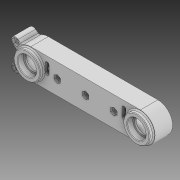
# Autodesk Inventor part: Scara1
Saved by Autodesk Inventor 2020 (Build 240168000, 168)
## iProperties
Created: 2020-07-24
Part Number: Scara1
Material: Generic
Document SubType Name: Modeling
Designer: DDeGo
Density: 1 g/cm^3
Appearance: Default
Author: DDeGo
Autodesk Inventor part; units mm, degrees
ref_plane "YZ Plane" through (0, 0, 0) normal (1, 0, 0) x (0, 1, 0)
ref_plane "XZ Plane" through (0, 0, 0) normal (0, 1, 0) x (-1, 0, 0)
ref_plane "XY Plane" through (0, 0, 0) normal (0, 0, 1) x (1, 0, 0)
sketch "Sketch1" plane through (0, 0, 0) normal (0, 0, 1) x (1, 0, 0)
  line L0 (0, 0) -> (97, 0) construction
  line L1 (0, -13) -> (97, -13)
  line L2 (97, 13) -> (0, 13)
  arc A0 (0, 13) -> (0, -13) centre (0, 0) ccw
  arc A1 (97, -13) -> (97, 13) centre (97, 0) ccw
  point P0 (48.5, 0)
  dimension "d0" = 97
  dimension "d1" = 13
  constraints: 8 end point, 4 point on circle, 4 tangent, 2 centre point, 1 horizontal, 1 midpoint, 1 parallel
  measures "d0" distance of L0.start L0.end
  measures "d1" radius of A0
extrude "Extrusion1" add sketch "Sketch1" along normal blind 3
sketch "Sketch2" plane through (0, 0, 0) normal (0, 0, -1) x (-1, 0, 0)
  line L0 (-97, 13) -> (0, 13) projected
  arc A0 (-97, 13) -> (-97, -13) centre (-97, 0) ccw projected
  line L1 (0, -13) -> (-97, -13) projected
  arc A1 (0, -13) -> (0, 13) centre (0, 0) ccw projected
  line L2 (0, 10) -> (-97, 10)
  arc A2 (-97, 10) -> (-97, -10) centre (-97, 0) ccw
  line L3 (-97, -10) -> (0, -10)
  arc A3 (0, -10) -> (0, 10) centre (0, 0) ccw
  point P0 (-94.4322, -13)
  dimension "d17" = 3
  constraints: 4 end point, 4 point on circle, 2 centre point, 1 point on line, 3 other
  measures "d17" distance between parallel lines of L2 L0
extrude "Extrusion2" add sketch "Sketch2" along normal blind 12.5
sketch "Sketch5" plane through (0, 0, 0) normal (0, 0, -1) x (-1, 0, 0)
  circle A0 centre (0, 0) radius 3
  arc A1 (-97, 13) -> (-97, -13) centre (-97, 0) ccw projected
  circle A2 centre (-97, 0) radius 3
  dimension "d14" = 6
  constraints: 2 centre point, 2 coincident, 1 equal radius
  measures "d14" diameter of A2
extrude "Extrusion5" cut sketch "Sketch5" against normal through all
sketch "Sketch6" plane through (0, 0, 3) normal (0, 0, 1) x (1, 0, 0)
  circle A0 centre (0, 0) radius 8.15
  circle A1 centre (0, 0) radius 11.65
  dimension "d18" = 16.3
  dimension "d19" = 3.5
  constraints: 2 centre point, 2 coincident
  measures "d18" diameter of A0
  measures "d19" radial gap between concentric circles of A1 A0
extrude "Extrusion6" add sketch "Sketch6" along normal blind 3.5
sketch "Sketch7" plane through (0, 0, 6.5) normal (0, 0, 1) x (1, 0, 0)
  circle A0 centre (0, 0) radius 8.15 projected
extrude "Extrusion7" cut sketch "Sketch7" against normal blind 5
chamfer "Chamfer1" distance 1 angle 45 1 edges at (-11.65, 0, 3)
sketch "Sketch8" plane through (0, 0, 1.5) normal (0, 0, 1) x (1, 0, 0)
  circle A0 centre (0, 0) radius 8.15 projected
  circle A1 centre (0, 0) radius 6.65
  dimension "d27" = 1.5
  constraints: 1 centre point
  measures "d27" radial gap between concentric circles of A0 A1
extrude "Extrusion8" cut sketch "Sketch8" against normal through all contours A1
sketch "Sketch9" plane through (0, 0, 0) normal (0, 0, -1) x (-1, 0, 0)
  circle A0 centre (-97, 0) radius 3 projected
  circle A1 centre (0, 0) radius 3 projected
  line L0 (-97, 0) -> (0, 0) construction
  circle A2 centre (-73.5, 0) radius 4
  circle A3 centre (-73.5, 0) radius 1.75
  circle A4 centre (-48.5, 0) radius 4
  circle A5 centre (-48.5, 0) radius 1.75
  circle A6 centre (-23.5, 0) radius 4
  circle A7 centre (-23.5, 0) radius 1.75
  dimension "d30" = 3.5
  dimension "d31" = 8
  dimension "d42" = 25
  dimension "d67" = 25
  constraints: 6 centre point, 4 equal radius, 3 coincident, 2 end point, 2 point on line, 1 horizontal, 1 midpoint
  measures "d30" diameter of A3
  measures "d31" diameter of A2
  measures "d42" distance of A4.centre A2.centre
  measures "d67" distance of A6.centre A4.centre
extrude "Extrusion9" add sketch "Sketch9" along normal up to surface (12.5 mm away) contours A2 | A4 | A6
sketch "Sketch10" plane through (0, 0, 0) normal (0, 1, 0) x (-1, 0, 0)
  line L0 (-69.5, 0) -> (-69.5, -12.5) projected
  line L1 (-52.5, 0) -> (-52.5, -12.5) projected
  line L2 (-44.5, 0) -> (-44.5, -12.5) projected
  line L3 (-27.5, 0) -> (-27.5, -12.5) projected
  line L4 (-69.5, -12.5) -> (-77.5, -12.5) projected
  line L5 (-69.5, -12.5) -> (-52.5, -12.5)
  line L6 (-44.5, -12.5) -> (-27.5, -12.5)
  line L7 (-44.5, 0) -> (-52.5, 0) projected
  line L8 (-27.5, 0) -> (-44.5, 0)
  line L9 (-69.5, 0) -> (-77.5, 0) projected
  line L10 (-52.5, 0) -> (-69.5, 0)
  line L11 (-69.5, -12.5) -> (-70.5, -12.5)
  line L12 (-70.5, -12.5) -> (-70.5, 0)
  line L13 (-69.5, 0) -> (-70.5, 0)
  line L14 (-44.5, -12.5) -> (-52.5, -12.5) projected
  line L15 (-52.5, -12.5) -> (-51.5, -12.5)
  line L16 (-51.5, -12.5) -> (-51.5, 0.1572)
  line L17 (-51.5, 0.1572) -> (-52.5, 0)
  line L18 (-44.5, 0) -> (-45.5, 0)
  line L19 (-44.5, -12.5) -> (-45.5, -12.5)
  line L20 (-45.5, -12.5) -> (-45.5, 0)
  line L21 (-27.5, -12.5) -> (-26.5, -12.5)
  line L22 (-26.5, -12.5) -> (-26.5, 0)
  line L23 (-19.5, 0) -> (-27.5, 0) projected
  line L24 (-26.5, 0) -> (-27.5, 0)
  line L25 (-27.5, 0) -> (-26.5, 0)
  circle A0 centre (-73.4335, -3.2498) radius 2
  circle A1 centre (-56.5768, -5.2498) radius 2
  circle A2 centre (-26.4602, -5.2498) radius 2
  circle A3 centre (-43.2818, -5.75) radius 2
  point P0 (0, 0)
  point P1 (-51.5, 0)
  dimension "d38" = 1
  dimension "d39" = 1
  dimension "d40" = 1
  dimension "d41" = 1
  dimension "d50" = 4
  dimension "d51" = 4
  dimension "d52" = 4
  dimension "d53" = 4
  constraints: 34 end point, 6 point on line, 5 perpendicular, 4 centre point, 4 collinear, 2 horizontal, 1 parallel
  measures "d38" distance between parallel lines of L3 L22
  measures "d39" distance between parallel lines of L2 L20
  measures "d40" distance between parallel lines of L1 L16
  measures "d41" distance between parallel lines of L0 L12
  measures "d50" diameter of A2
  measures "d51" diameter of A1
  measures "d52" diameter of A0
  measures "d53" diameter of A3
extrude "Extrusion10" add sketch "Sketch10" along normal mid plane 3 contours L10 L1 L5 L0 | L0 L4 L12 L9 | L7 L16 L14 L1 | L7 L2 A3 L14 L20 | L8 L3 A2 L6 L2 A3 | L2 A3 | L23 L22 A2 L3 | L3 A2 L22 L21 | A2 L22 L3 picked at (-44.7432, -5.9013)
pattern_linear "Rectangular Pattern1" count 2 spacing 97 along (1, 0, 0) of "Extrusion8", "Extrusion6", "Chamfer1", "Extrusion7"
sketch "Sketch11" plane through (0, 0, 3) normal (0, 0, 1) x (1, 0, 0)
  circle A0 centre (97, 0) radius 4.8676
  line L0 (97, 0) -> (82.5, 0) construction
  line L1 (82.5, 0) -> (82.5, 7) construction
  line L2 (84.2, 0) -> (84.2, 7)
  line L3 (80.8, 7) -> (80.8, 0)
  arc A1 (80.8, 0) -> (84.2, 0) centre (82.5, 0) ccw
  arc A2 (84.2, 7) -> (80.8, 7) centre (82.5, 7) ccw
  line L4 (0, 13) -> (97, 13) projected
  line L5 (48.5, 13) -> (48.5, -13) construction
  line L6 (97, -13) -> (0, -13) projected
  line L7 (14.5, 0) -> (14.5, 7) construction
  line L8 (12.8, 0) -> (12.8, 7)
  line L9 (16.2, 7) -> (16.2, 0)
  arc A3 (12.8, 0) -> (16.2, 0) centre (14.5, 0) ccw
  arc A4 (16.2, 7) -> (12.8, 7) centre (14.5, 7) ccw
  circle A5 centre (97, 0) radius 8.15 projected
  point P0 (0, 0)
  dimension "d47" = 14.5
  dimension "d65" = 1.7
  dimension "d66" = 7
  constraints: 20 end point, 8 point on circle, 6 symmetric about line, 5 centre point, 4 tangent, 2 midpoint, 1 concentric, 1 horizontal, 1 parallel, 1 vertical, 2 other
  measures "d47" distance of L0.end L0.start
  measures "d65" radius of A2
  measures "d66" distance of L0.end L1.end
extrude "Extrusion11" cut sketch "Sketch11" against normal up to surface (3 mm away) contours A1 L3 A2 L2 | L8 A4 L9 A3
sketch "Sketch14" plane through (73.5, 0, 0) normal (0, 0, -1) x (-1, 0, 0)
  circle A0 centre (50, 0) radius 1.75 projected
  circle A1 centre (25, 0) radius 1.75 projected
  circle A2 centre (0, 0) radius 1.75 projected
  point P0 (73.5, 0)
extrude "Extrusion13" cut sketch "Sketch14" against normal through all
chamfer "Chamfer2" distance 0.5 angle 45 4 edges at (-8.15, 0, 6.5) (-11.65, 0, 6.5) (88.85, 0, 6.5) (85.35, 0, 6.5)
sketch "Sketch16" plane through (0, 0, -12.5) normal (0, 0, -1) x (-1, 0, 0)
  circle A0 centre (13.4374, -10) radius 1.6
  arc A1 (11.1985, -13.0084) -> (15.6762, -6.9916) centre (13.4374, -10) ccw
  arc A2 (0, -13) -> (0, 13) centre (0, 0) ccw projected
  line L0 (0, 0) -> (13, 0) construction
  line L1 (15.6762, -6.9916) -> (12.2245, -4.4229)
  line L2 (12.2245, -4.4229) -> (7.7469, -10.4396)
  line L3 (7.7469, -10.4396) -> (11.1985, -13.0084)
  circle A3 centre (13.4374, 10) radius 1.6
  arc A4 (15.6762, 6.9916) -> (11.1985, 13.0084) centre (13.4374, 10) ccw
  line L4 (15.6762, 6.9916) -> (12.2245, 4.4229)
  line L5 (12.2245, 4.4229) -> (7.7469, 10.4396)
  line L6 (7.7469, 10.4396) -> (11.1985, 13.0084)
  point P0 (7.7469, 10.4396)
  point P1 (12.2245, 4.4229)
  dimension "d68" = 7.5
  dimension "d69" = 3.2
  dimension "d70" = 10
  constraints: 14 end point, 7 point on circle, 6 symmetric about line, 4 centre point, 3 tangent, 2 coincident, 2 perpendicular, 2 other
  measures "d68" diameter of A1
  measures "d69" diameter of A0
  measures "d70" vertical distance of point (0, 0) A0.centre
extrude "Extrusion15" add sketch "Sketch16" against normal up to surface (15.5 mm away) contours L3 A2 L1 A1 | A2 L6 A4 L4
sketch "Sketch15" plane through (0, 0, 3) normal (0, 0, 1) x (1, 0, 0)
  circle A0 centre (73.5, 0) radius 1.75 projected
  line L0 (73.5, -3.3486) -> (70.6, -1.6743)
  line L1 (70.6, -1.6743) -> (70.6, 1.6743)
  line L2 (70.6, 1.6743) -> (73.5, 3.3486)
  line L3 (73.5, 3.3486) -> (76.4, 1.6743)
  line L4 (76.4, 1.6743) -> (76.4, -1.6743)
  line L5 (76.4, -1.6743) -> (73.5, -3.3486)
  circle A1 centre (48.5, 0) radius 1.75 projected
  line L6 (48.5, -3.3486) -> (45.6, -1.6743)
  line L7 (45.6, -1.6743) -> (45.6, 1.6743)
  line L8 (45.6, 1.6743) -> (48.5, 3.3486)
  line L9 (48.5, 3.3486) -> (51.4, 1.6743)
  line L10 (51.4, 1.6743) -> (51.4, -1.6743)
  line L11 (51.4, -1.6743) -> (48.5, -3.3486)
  circle A2 centre (23.5, 0) radius 1.75 projected
  line L12 (23.5, -3.3486) -> (20.6, -1.6743)
  line L13 (20.6, -1.6743) -> (20.6, 1.6743)
  line L14 (20.6, 1.6743) -> (23.5, 3.3486)
  line L15 (23.5, 3.3486) -> (26.4, 1.6743)
  line L16 (26.4, 1.6743) -> (26.4, -1.6743)
  line L17 (26.4, -1.6743) -> (23.5, -3.3486)
  circle A3 centre (-13.4374, 10) radius 1.6 projected
  line L18 (-11.4382, 12.6864) -> (-10.1113, 9.6118)
  line L19 (-10.1113, 9.6118) -> (-12.1105, 6.9255)
  line L20 (-12.1105, 6.9255) -> (-15.4365, 7.3136)
  line L21 (-15.4365, 7.3136) -> (-16.7634, 10.3882)
  line L22 (-16.7634, 10.3882) -> (-14.7642, 13.0745)
  line L23 (-14.7642, 13.0745) -> (-11.4382, 12.6864)
  circle A4 centre (-13.4374, -10) radius 1.6 projected
  line L24 (-11.4382, -12.6864) -> (-14.7642, -13.0745)
  line L25 (-14.7642, -13.0745) -> (-16.7634, -10.3882)
  line L26 (-16.7634, -10.3882) -> (-15.4365, -7.3136)
  line L27 (-15.4365, -7.3136) -> (-12.1105, -6.9255)
  line L28 (-12.1105, -6.9255) -> (-10.1113, -9.6118)
  line L29 (-10.1113, -9.6118) -> (-11.4382, -12.6864)
  line L30 (-11.1985, 13.0084) -> (-7.7469, 10.4396) projected
  line L31 (-7.7469, 10.4396) -> (-12.2245, 4.4229) construction
  line L32 (-15.6762, -6.9916) -> (-12.2245, -4.4229) projected
  line L33 (-7.7469, -10.4396) -> (-11.1985, -13.0084) projected
  line L34 (-12.2245, -4.4229) -> (-7.7469, -10.4396) construction
  point P0 (0, 0)
  dimension "d59" = 5.8
  constraints: 64 end point, 5 coincident, 4 equal length, 3 vertical, 2 parallel, 1 perpendicular, 65 other
  measures "d59" distance between parallel lines of L1 L4
extrude "Extrusion14" cut sketch "Sketch15" against normal blind 2 contours A0 | L0 L1 L2 L3 L4 L5 | A1 | L6 L7 L8 L9 L10 L11 | A2 | L12 L13 L14 L15 L16 L17 | L18 L19 L20 L21 L22 L23 | L24 L25 L26 L27 L28 L29
fillet "Fillet1" radius 2 4 edges at (-7.7469, 10.4396, -4.75) (-12.2245, -4.4229, -4.75) (-12.2245, 4.4229, -4.75) (-7.7469, -10.4396, -4.75)
equation "\"d67\" = d42"
equation "\"d45\" = d0"
body "Solid1"
